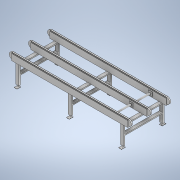
# Autodesk Inventor part: banda transportadora
Saved by Autodesk Inventor 2021 (Build 250183000, 183)
## iProperties
Created: 2021-07-31
Part Number: banda transportadora
Material: Generic
Document SubType Name: Modeling
Designer: juanc
Density: 1 g/cm^3
Appearance: Default
Author: juanc
Autodesk Inventor part; units mm, degrees
ref_plane "YZ Plane" through (0, 0, 0) normal (1, 0, 0) x (0, 1, 0)
ref_plane "XZ Plane" through (0, 0, 0) normal (0, 1, 0) x (-1, 0, 0)
sketch "Sketch1" plane through (0, 0, 0) normal (0, 0, 1) x (1, 0, 0)
  line L0 (-1500, -80) -> (1500, -80)
  line L1 (1500, -80) -> (1500, 80)
  line L2 (1500, 80) -> (-1500, 80)
  line L3 (-1500, 80) -> (-1500, -80)
  line L4 (-1500, -80) -> (1500, 80) construction
  line L5 (1500, -80) -> (-1500, 80) construction
  point P0 (0, 0)
  dimension "d0" = 3000
  dimension "d1" = 160
  constraints: 12 end point, 2 midpoint, 2 parallel, 1 horizontal, 1 perpendicular
  measures "d0" distance of L2.end L1.end
  measures "d1" distance of L1.end L0.end
extrude "Extrusion1" add sketch "Sketch1" against normal blind 30
sketch "Sketch2" plane through (1500, -80, 0) normal (1, 0, 0) x (0, 0, -1)
  line L0 (30, 160) -> (30, 0) construction
  line L1 (30, 160) -> (15, 160)
  line L2 (15, 160) -> (15, 22.332)
  line L3 (15, 22.332) -> (30, 22.332)
  line L4 (30, 22.332) -> (30, 160)
  line L5 (0, 0) -> (30, 0) construction
  point P0 (0, 80)
  dimension "d4" = 15
  dimension "d5" = 22.332
  constraints: 8 end point, 2 parallel, 1 horizontal, 1 perpendicular
  measures "d4" distance of L3.end L2.end
  measures "d5" distance between parallel lines of L5 L3
extrude "Extrusion2" cut sketch "Sketch2" against normal blind 3000
sketch "Sketch3" plane through (-1500, 80, 0) normal (0, 1, 0) x (1, 0, 0)
  line L0 (3000, 0) -> (0, 0) construction
  line L1 (3000, 0) -> (3000, 15) projected
  line L2 (3000, 15) -> (0, 15)
  line L3 (0, 15) -> (0, 7.5)
  line L4 (0, 7.5) -> (3000, 7.5)
  line L5 (3000, 7.5) -> (3000, 15)
  point P0 (1500, 0)
  dimension "d8" = 3000
  dimension "d9" = 7.5
  constraints: 8 end point, 2 parallel, 1 horizontal, 1 perpendicular
  measures "d8" distance of L4.end L3.end
  measures "d9" distance of L3.end L2.end
extrude "Extrusion3" add sketch "Sketch3" along normal blind 15
sketch "Sketch4" plane through (1500, -57.668, -15) normal (0, 0, -1) x (-1, 0, 0)
  line L0 (0, 152.668) -> (3000, 152.668) construction
  line L1 (0, 157.668) -> (3000, 157.668)
  line L2 (0, 0) -> (3000, 0) projected
  arc A0 (0, 157.668) -> (0, 0) centre (0, 78.834) ccw
  arc A1 (3000, 0) -> (3000, 157.668) centre (3000, 78.834) ccw
  point P0 (1500, 57.668)
  dimension "d13" = 5
  dimension "d14" = 78.834
  dimension "d15" = 3000
  constraints: 4 point on circle, 2 centre point, 2 end point, 2 tangent, 1 horizontal
  measures "d13" distance between parallel lines of L0 L1
  measures "d14" radius of A0
  measures "d15" distance of L1.start L1.end
extrude "Extrusion4" add sketch "Sketch4" along normal blind 15
mirror "Mirror1" about plane through (0, 0, -30) normal (0, 0, -1) of "Extrusion1", "Extrusion4", "Extrusion3"
pattern_linear "Rectangular Pattern1" count 3 spacing 495.5 along (0, 0, -1)
sketch "Sketch5" plane through (-1500, -80, -991) normal (0, -1, 0) x (1, 0, 0)
  line L0 (0, -60) -> (3000, -60) construction
  line L1 (2890, -60) -> (2810, -60)
  line L2 (2810, -60) -> (2810, -20)
  line L3 (2810, -20) -> (2890, -20)
  line L4 (2890, -20) -> (2890, -60)
  point P0 (1500, 991)
  dimension "d21" = 80
  dimension "d22" = 40
  dimension "d23" = 110
  constraints: 8 end point, 2 parallel, 1 horizontal, 1 perpendicular, 1 point on line
  measures "d21" distance of L2.end L3.end
  measures "d22" distance of L1.end L2.end
  measures "d23" distance from line of L0.end L4
extrude "Extrusion5" add sketch "Sketch5" along normal blind 470
sketch "Sketch6" plane through (-1500, -550, -991) normal (0, -1, 0) x (1, 0, 0)
  line L0 (2810, -60) -> (2890, -60) projected
  line L1 (2890, -60) -> (2890, -20) projected
  circle A0 centre (2850, -40) radius 10
  point P0 (1500, 991)
  dimension "d26" = 20
  dimension "d27" = 40
  dimension "d28" = 20
  constraints: 1 centre point, 1 coincident
  measures "d26" distance from line of L0 point (2850, -40)
  measures "d27" distance from line of L1 point (2850, -40)
  measures "d28" diameter of A0
extrude "Extrusion6" add sketch "Sketch6" along normal blind 45
sketch "Sketch7" plane through (1350, -595, -1031) normal (0, -1, 0) x (1, 0, 0)
  line L0 (40, 30) -> (-35, 30)
  line L1 (-35, 30) -> (-35, -70)
  line L2 (-35, -70) -> (40, -70)
  line L3 (40, -70) -> (40, 30)
  circle A0 centre (0, 0) radius 10 construction
  point P0 (-1350, 1031)
  dimension "d31" = 100
  dimension "d32" = 75
  dimension "d33" = 30
  dimension "d34" = 35
  constraints: 8 end point, 2 parallel, 1 horizontal, 1 perpendicular
  measures "d31" distance of L2.end L0.start
  measures "d32" distance of L0.start L0.end
  measures "d33" distance from line of L0 A0.centre
  measures "d34" distance from line of L1 A0.centre
extrude "Extrusion7" add sketch "Sketch7" along normal blind 5
ref_plane "Work Plane1" through (-1500, -80, -991) normal (0, -1, 0) x (1, 0, 0)
split body "Split1" result two bodies by plane through (-1500, -80, -991) normal (0, -1, 0) first body at (1336.6667, -236.6667, -1050.5)
sketch "Sketch8" plane through (1310, -550, -1011) normal (0, 0, 1) x (1, 0, 0)
  line L0 (0, 470) -> (80, 470)
  line L1 (80, 470) -> (80, 442)
  line L2 (80, 442) -> (0, 442)
  line L3 (0, 442) -> (0, 470)
  line L4 (0, 470) -> (0, 0) construction
  line L5 (0, 249) -> (80, 249)
  line L6 (80, 249) -> (80, 221)
  line L7 (80, 221) -> (0, 221)
  line L8 (0, 221) -> (0, 249)
  point P0 (-1310, 550)
  dimension "d41" = 80
  dimension "d42" = 28
  dimension "d43" = 80
  dimension "d44" = 28
  dimension "d45" = 193
  constraints: 16 end point, 4 parallel, 2 horizontal, 2 perpendicular, 1 point on line
  measures "d41" distance of L1.end L2.end
  measures "d42" distance of L0.end L1.end
  measures "d43" distance of L6.end L7.end
  measures "d44" distance of L5.end L6.end
  measures "d45" distance between parallel lines of L5 L2
extrude "Extrusion8" add sketch "Sketch8" along normal blind 485.5 bodies 2
pattern_linear "Rectangular Pattern3" count 3 spacing 1350 along (-1, 0, 0) bodies 2
mirror "Mirror2" about plane through (1350, -315, -525.5) normal (0, 0, 1) bodies 2
sketch "Sketch9" plane through (-1500, 80, -991) normal (0, 0, 1) x (1, 0, 0)
  line L0 (2550, -30) -> (2650, -30)
  line L1 (2650, -30) -> (2650, -130)
  line L2 (2650, -130) -> (2550, -130)
  line L3 (2550, -130) -> (2550, -30)
  line L4 (3000, 0) -> (0, 0) projected
  line L5 (3000, -160) -> (3000, 0) projected
  point P0 (1500, -80)
  dimension "d51" = 100
  dimension "d52" = 100
  dimension "d53" = 30
  dimension "d54" = 350
  constraints: 8 end point, 2 parallel, 1 horizontal, 1 perpendicular
  measures "d51" distance of L1.end L2.end
  measures "d52" distance of L0.end L1.end
  measures "d53" distance between parallel lines of L4 L0
  measures "d54" distance between parallel lines of L5 L1
extrude "Extrusion9" add sketch "Sketch9" along normal blind 10 bodies 3
sketch "Sketch10" plane through (-1500, 80, -981) normal (0, 0, 1) x (1, 0, 0)
  circle A0 centre (2600, -80) radius 24
  line L0 (2650, -130) -> (2650, -30) construction
  line L1 (2650, -30) -> (2550, -30) construction
  point P0 (1500, -80)
  dimension "d57" = 48
  dimension "d58" = 50
  dimension "d59" = 50
  constraints: 1 centre point
  measures "d57" diameter of A0
  measures "d58" distance from line of L0 A0.centre
  measures "d59" distance from line of L1 A0.centre
extrude "Extrusion10" add sketch "Sketch10" along normal blind 10 bodies 3
sketch "Sketch11" plane through (1100, 0, -971) normal (0, 0, 1) x (1, 0, 0)
  circle A0 centre (0, 0) radius 20
  point P0 (-1100, 0)
  dimension "d62" = 40
  constraints: 1 centre point
  measures "d62" diameter of A0
extrude "Extrusion11" add sketch "Sketch11" along normal blind 395.5 bodies 3
sketch "Sketch12" plane through (1100, 0, -575.5) normal (0, 0, 1) x (1, 0, 0)
  circle A0 centre (0, 0) radius 24
  point P0 (-1100, 0)
  dimension "d65" = 48
  constraints: 1 centre point
  measures "d65" diameter of A0
extrude "Extrusion12" add sketch "Sketch12" along normal blind 10 bodies 3
sketch "Sketch13" plane through (1100, 0, -565.5) normal (0, 0, 1) x (1, 0, 0)
  line L0 (50, -50) -> (-50, -50)
  line L1 (-50, -50) -> (-50, 50)
  line L2 (-50, 50) -> (50, 50)
  line L3 (50, 50) -> (50, -50)
  circle A0 centre (0, 0) radius 20 construction
  line L4 (50, -50) -> (-50, 50) construction
  line L5 (-50, -50) -> (50, 50) construction
  point P0 (-1100, 0)
  dimension "d68" = 100
  dimension "d69" = 100
  constraints: 12 end point, 2 midpoint, 2 parallel, 1 horizontal, 1 perpendicular
  measures "d68" distance of L1.end L2.end
  measures "d69" distance of L0.end L1.end
extrude "Extrusion13" add sketch "Sketch13" along normal blind 10 bodies 3
sketch "Sketch14" plane through (-1500, 80, -495.5) normal (0, 0, 1) x (1, 0, 0)
  line L0 (2650, -130) -> (2550, -130)
  line L1 (2550, -130) -> (2550, -30)
  line L2 (2550, -30) -> (2650, -30)
  line L3 (2650, -30) -> (2650, -130)
  line L4 (2650, -130) -> (2550, -30) construction
  line L5 (2550, -130) -> (2650, -30) construction
  line L6 (3000, 0) -> (0, 0) construction
  line L7 (3000, -160) -> (3000, 0) projected
  point P0 (1500, -80)
  point P1 (2600, -80)
  dimension "d72" = 100
  dimension "d73" = 100
  dimension "d74" = 30
  dimension "d75" = 350
  constraints: 12 end point, 2 midpoint, 2 parallel, 1 horizontal, 1 perpendicular
  measures "d72" distance of L1.end L2.end
  measures "d73" distance of L0.end L1.end
  measures "d74" distance between parallel lines of L6 L2
  measures "d75" distance between parallel lines of L7 L3
extrude "Extrusion14" add sketch "Sketch14" along normal blind 10 bodies 3
sketch "Sketch15" plane through (-1500, 80, -485.5) normal (0, 0, 1) x (1, 0, 0)
  circle A0 centre (2600, -80) radius 24
  line L0 (2650, -30) -> (2550, -30) construction
  line L1 (2550, -30) -> (2550, -130) construction
  point P0 (1500, -80)
  dimension "d78" = 48
  dimension "d79" = 50
  dimension "d80" = 50
  constraints: 1 centre point
  measures "d78" diameter of A0
  measures "d79" distance from line of L0 A0.centre
  measures "d80" distance from line of L1 A0.centre
extrude "Extrusion15" add sketch "Sketch15" along normal blind 10 bodies 3
sketch "Sketch16" plane through (1100, 0, -475.5) normal (0, 0, 1) x (1, 0, 0)
  circle A0 centre (0, 0) radius 20
  point P0 (-1100, 0)
  dimension "d83" = 40
  constraints: 1 centre point
  measures "d83" diameter of A0
extrude "Extrusion16" add sketch "Sketch16" along normal blind 395.5 bodies 3
sketch "Sketch17" plane through (1100, 0, -80) normal (0, 0, 1) x (1, 0, 0)
  circle A0 centre (0, 0) radius 24
  point P0 (-1100, 0)
  dimension "d86" = 48
  constraints: 1 centre point
  measures "d86" diameter of A0
extrude "Extrusion17" add sketch "Sketch17" along normal blind 10 bodies 3
sketch "Sketch18" plane through (1100, 0, -70) normal (0, 0, 1) x (1, 0, 0)
  line L0 (50, -50) -> (-50, -50)
  line L1 (-50, -50) -> (-50, 50)
  line L2 (-50, 50) -> (50, 50)
  line L3 (50, 50) -> (50, -50)
  line L4 (50, -50) -> (-50, 50) construction
  line L5 (-50, -50) -> (50, 50) construction
  point P0 (-1100, 0)
  point P1 (0, 0)
  dimension "d89" = 100
  dimension "d90" = 100
  constraints: 12 end point, 2 midpoint, 2 parallel, 1 horizontal, 1 perpendicular
  measures "d89" distance of L1.end L2.end
  measures "d90" distance of L0.end L1.end
extrude "Extrusion18" add sketch "Sketch18" along normal blind 10 bodies 3
body "Solid2"
body "Solid3"
